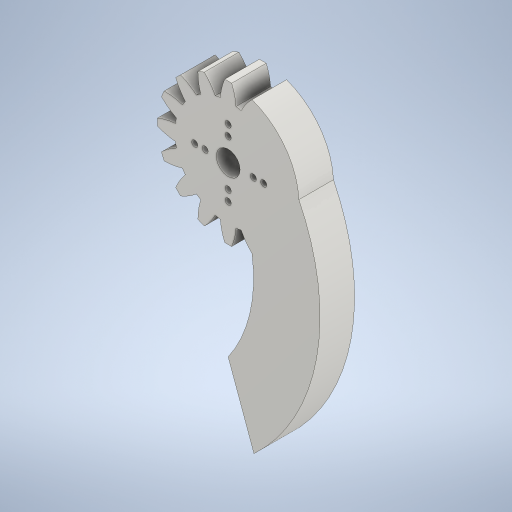
# Autodesk Inventor part: Spur Gear2
Saved by Autodesk Inventor 2024 (Build 280153000, 153)
## iProperties
CustomPartVersion: 0
Created: 2023-09-24
Part Number: Spur Gear2
Material: Steel
Document SubType Name: Modeling
Designer: jebes windows
Categories: <?xml version="1.0" encoding="UTF-16"?> <MemberInstance><Categories><FamilyTemplate><FamilyTemplateParameter ValueType="xs:double" Id="1" ObjectReferenceKey="da_z" ObjectType="kUserParameterObject"/><FamilyTemplateParameter ValueType="xs:double" Id="2" ObjectReferenceKey="da_b" ObjectType="kUserParameterObject"/><FamilyTemplateParameter ValueType="xs:double" Id="3" ObjectReferenceKey="da_beta" ObjectType="kUserParameterObject"/><FamilyTemplateParameter ValueType="xs:double" Id="4" ObjectReferenceKey="da_da" ObjectType="kUserParameterObject"/><FamilyTemplateParameter ValueType="xs:double" Id="5" ObjectReferenceKey="da_aw" ObjectType="kUserParameterObject"/><FamilyTemplateParameter ValueType="xs:string" Id="6" ObjectReferenceKey="EAIAABAAAACIAQAAAAAAAIAAAAAAAAAA" ObjectType="83910656" SubObjectId="SurfaceGeometry"/></FamilyTemplate><ParamToTemplateMap><ParamToTemplate CategoryParameter="//CategoryParameter[@InternalName='046C89C9-8512-4d59-83FE-43B91F4F132A']" TemplateParameter="1"/><ParamToTemplate CategoryParameter="//CategoryParameter[@InternalName='2552DF32-E462-4b46-AEBF-C6C7768E72AC']" TemplateParameter="2"/><ParamToTemplate CategoryParameter="//CategoryParameter[@InternalName='C9EE641D-15FC-4fae-A226-E94C4372FDD7']" TemplateParameter="3"/><ParamToTemplate><ParamToTemplate CategoryParameter="//CategoryParameter[@InternalName='00B6519A-459B-49c7-AD84-2E56D39A5744']" ConstantValue="0.102382"/></ParamToTemplate><ParamToTemplate><ParamToTemplate CategoryParameter="//CategoryParameter[@InternalName='04B31F0E-C7A6-4894-AA32-9629BEFACF47']" ConstantValue="1.000000"/></ParamToTemplate><ParamToTemplate><ParamToTemplate CategoryParameter="//CategoryParameter[@InternalName='43CBEC2E-7847-49e7-A936-2F7889FCB2D9']" ConstantValue="0.250000"/></ParamToTemplate><ParamToTemplate><ParamToTemplate CategoryParameter="//CategoryParameter[@InternalName='B1EFC894-105D-4ebd-86BF-FA20ED196853']" ConstantValue="0.302500"/></ParamToTemplate><ParamToTemplate><ParamToTemplate CategoryParameter="//CategoryParameter[@InternalName='51175063-3D10-4879-93E8-6246FE8B403D']" ConstantValue="2060000000.000000"/></ParamToTemplate><ParamToTemplate><ParamToTemplate CategoryParameter="//CategoryParameter[@InternalName='A3A52E27-4454-46a9-B0BD-C932399B70AF']" ConstantValue="0.300000"/></ParamToTemplate><ParamToTemplate><ParamToTemplate CategoryParameter="//CategoryParameter[@InternalName='91B76062-C214-41d9-B1B9-14D2AB99603D']" ConstantValue="0.150000"/></ParamToTemplate><ParamToTemplate><ParamToTemplate CategoryParameter="//CategoryParameter[@InternalName='374E806E-8B8A-4dda-A9AA-1039D6500AD2']" ConstantValue="6.666667"/></ParamToTemplate><ParamToTemplate><ParamToTemplate CategoryParameter="//CategoryParameter[@InternalName='2D373A89-B862-43d6-8D0B-0CBF12AB9F6C']" ConstantValue="0.349066"/></ParamToTemplate><ParamToTemplate CategoryParameter="//CategoryParameter[@InternalName='37777632-D6A2-4fac-9D53-DB8ACD95C989']" TemplateParameter="4"/><ParamToTemplate CategoryParameter="//CategoryParameter[@InternalName='FD1017F1-B727-4f7e-9707-0F86F1FF9423']" TemplateParameter="5"/><ParamToTemplate><ParamToTemplate CategoryParameter="//CategoryParameter[@InternalName='9E1B4470-B2D3-4ff1-B813-535BB4CDF51A']" ConstantValue="3520000.000000"/></ParamToTemplate><ParamToTemplate><ParamToTemplate CategoryParameter="//CategoryParameter[@InternalName='F8452263-BFF6-458c-9FB1-07C4B99E95CD']" ConstantValue="11400000.000000"/></ParamToTemplate><ParamToTemplate><ParamToTemplate CategoryParameter="//CategoryParameter[@InternalName='3E3BB259-FD49-497f-8171-6EBC954A3479']" ConstantValue="2.000000"/></ParamToTemplate><ParamToTemplate CategoryParameter="//CategoryParameter[@InternalName='27C3BAF2-7550-4e4b-AE2C-0DB134B7D9B7']" TemplateParameter="6"/></ParamToTemplateMap><Category DisplayName="Gear" InternalName="DC85795E-93AB-48d5-8EEE-5A27447B64BD" Mnemonic="Gear"><CategoryParameter DisplayName="z" InternalName="046C89C9-8512-4d59-83FE-43B91F4F132A" Mnemonic="z"/><CategoryParameter DisplayName="b" InternalName="2552DF32-E462-4b46-AEBF-C6C7768E72AC" Mnemonic="b"/><CategoryParameter DisplayName="||b|" InternalName="C9EE641D-15FC-4fae-A226-E94C4372FDD7" Mnemonic="beta"/><CategoryParameter DisplayName="x" InternalName="00B6519A-459B-49c7-AD84-2E56D39A5744" Mnemonic="x"/><CategoryParameter DisplayName="a*" InternalName="04B31F0E-C7A6-4894-AA32-9629BEFACF47" Mnemonic="a"/><CategoryParameter DisplayName="c*" InternalName="43CBEC2E-7847-49e7-A936-2F7889FCB2D9" Mnemonic="c"/><CategoryParameter DisplayName="r|.f|*" InternalName="B1EFC894-105D-4ebd-86BF-FA20ED196853" Mnemonic="rf"/><CategoryParameter DisplayName="E" InternalName="51175063-3D10-4879-93E8-6246FE8B403D" Mnemonic="E"/><CategoryParameter DisplayName="||m|" InternalName="A3A52E27-4454-46a9-B0BD-C932399B70AF" Mnemonic="mi"/><Category DisplayName="SpurGear" InternalName="26C5A22E-A91E-4dfd-A3B3-23CCAFAE1764" Mnemonic="SpurGear"><CategoryParameter DisplayName="m" InternalName="91B76062-C214-41d9-B1B9-14D2AB99603D" Mnemonic="m"/><CategoryParameter DisplayName="P" InternalName="374E806E-8B8A-4dda-A9AA-1039D6500AD2" Mnemonic="PP"/><CategoryParameter DisplayName="||a|" InternalName="2D373A89-B862-43d6-8D0B-0CBF12AB9F6C" Mnemonic="alpha"/><CategoryParameter DisplayName="d|.a|" InternalName="37777632-D6A2-4fac-9D53-DB8ACD95C989" Mnemonic="da"/><CategoryParameter DisplayName="a|.w|" InternalName="FD1017F1-B727-4f7e-9707-0F86F1FF9423" Mnemonic="aw"/><CategoryParameter DisplayName="||s||.Flim|" InternalName="9E1B4470-B2D3-4ff1-B813-535BB4CDF51A" Mnemonic="sFlim"/><CategoryParameter DisplayName="||s||.Hlim|" InternalName="F8452263-BFF6-458c-9FB1-07C4B99E95CD" Mnemonic="sHlim"/><CategoryParameter DisplayName="type" InternalName="3E3BB259-FD49-497f-8171-6EBC954A3479" Mnemonic="type"/><CategoryParameter DisplayName="PitchDiameter" InternalName="27C3BAF2-7550-4e4b-AE2C-0DB134B7D9B7" Mnemonic="IDS_PITCHDIAM"/></Category></Category></Categories></MemberInstance>
Density: 1 g/cm^3
Appearance: Steel
d16: 23,400 mm
d17: 0,000 mm
d41: 0,000 mm
d43: 23,400 mm
d46: 23,400 mm
d47: 0,000 mm
d48: 0,000 mm
Author: jebes windows
## iProperties of the stored document Spur Gear21_3DPrint.ipt
Created: 2023-09-24
Part Number: Spur Gear21_3DPrint
Material: Generic
Document SubType Name: Modeling
Designer: jebes windows
Density: 1 g/cm^3
Appearance: Default
Author: jebes windows
Autodesk Inventor part; units mm, degrees
ref_plane "YZ Plane" through (0, 0, 0) normal (1, 0, 0) x (0, 1, 0)
ref_plane "XZ Plane" through (0, 0, 0) normal (0, 1, 0) x (-1, 0, 0)
ref_plane "XY Plane" through (0, 0, 0) normal (0, 0, 1) x (1, 0, 0)
sketch "Sketch1" plane through (0, 0, 0) normal (0, 0, 1) x (1, 0, 0)
  circle A0 centre (0, 0) radius 13.65
  dimension "d0" = 27.3
  constraints: 1 centre point
  measures "d0" diameter of A0
extrude "Extrusion1" add sketch "Sketch1" along normal blind 6.6667
ref_plane "Work Plane2" through (0, 0, 3.3333) normal (0, 0, 1) x (1, 0, 0)
sketch "Sketch2" plane through (0, 0, 0) normal (0, 0, -1) x (-1, 0, 0)
  circle A0 centre (0, 0) radius 13.65 projected
  circle A1 centre (0, 0) radius 12
  dimension "d3" = 24
  constraints: 1 centre point, 1 coincident
  measures "d3" diameter of A1
surface extrude "Pitch Diameter" sketch "Sketch2" against normal through all shown no curves A1
ref_plane "Work Plane8" through (0, 0, 0) normal (0.9807853, 0.1950903, 0) x (0, 0, 1)
ref_plane "Work Plane9" through (0, 0, 0) normal (1, 0, 0) x (0, 1, 0)
spur gear teeth "Spur Gear" teeth 16 pitch diameter 24 tip diameter 27.3 root diameter 20.5571 face width 10 start plane through (0, 0, 0) normal (0, 0, -1) x (-1, 0, 0)
sketch "Sketch3" plane through (0, 0, 0) normal (0, 0, -1) x (-1, 0, 0)
  line L0 (1.9, -6.45) -> (1.9, -2.8797) projected
  arc A0 (1.9, -2.8797) -> (2.2091, -2.65) centre (0, 0) ccw projected
  line L1 (2.2091, -2.65) -> (14.1591, -1.997) projected
  arc A1 (14.1591, -1.997) -> (14.1591, 1.997) centre (14.05, 0) ccw projected
  line L2 (14.1591, 1.997) -> (2.2091, 2.65) projected
  arc A2 (2.2091, 2.65) -> (1.9, 2.8797) centre (0, 0) ccw projected
  line L3 (1.9, 2.8797) -> (1.9, 6.45) projected
  arc A3 (1.9, 6.45) -> (-1.9, 6.45) centre (0, 6.45) ccw projected
  line L4 (-1.9, 6.45) -> (-1.9, 3.2953) projected
  line L5 (-1.9, 3.2953) -> (-16.6263, 1.9922) projected
  arc A4 (-16.6263, 1.9922) -> (-16.6263, -1.9922) centre (-16.45, 0) ccw projected
  line L6 (-16.6263, -1.9922) -> (-1.9, -3.2953) projected
  line L7 (-1.9, -3.2953) -> (-1.9, -6.45) projected
  arc A5 (-1.9, -6.45) -> (1.9, -6.45) centre (0, -6.45) ccw projected
  circle A6 centre (-14.85, 0) radius 0.6 projected
  circle A7 centre (-16.85, 0) radius 0.6 projected
  circle A8 centre (-12.85, 0) radius 0.6 projected
  circle A9 centre (-10.85, 0) radius 0.6 projected
  circle A10 centre (-8.85, 0) radius 0.6 projected
  circle A11 centre (-6.85, 0) radius 0.6 projected
  circle A12 centre (-4.85, 0) radius 0.6 projected
  circle A13 centre (4.45, 0) radius 0.6 projected
  circle A14 centre (6.45, 0) radius 0.6 projected
  circle A15 centre (8.45, 0) radius 0.6 projected
  circle A16 centre (10.45, 0) radius 0.6 projected
  circle A17 centre (14.45, 0) radius 0.6 projected
  circle A18 centre (12.45, 0) radius 0.6 projected
  circle A19 centre (0, 0) radius 2.3 projected
  circle A20 centre (0, -4.45) radius 0.6 projected
  circle A21 centre (0, -6.45) radius 0.6 projected
  circle A22 centre (0, 4.45) radius 0.6 projected
  circle A23 centre (0, 6.45) radius 0.6 projected
  point P0 (0, 0)
extrude "Extrusion2" cut sketch "Sketch3" against normal blind 10 contours A11 | A12 | A13 | A14 | A19 | A20 | A21 | A22 | A23
sketch "Sketch4" plane through (0, 0, 6.6667) normal (0, 0, 1) x (1, 0, 0)
  circle A0 centre (0, 0) radius 2.3 projected
  circle A1 centre (0, 6.45) radius 0.6 projected
  circle A2 centre (0, -4.45) radius 0.6 projected
  circle A3 centre (-4.45, 0) radius 0.6 projected
  circle A4 centre (6.85, 0) radius 0.6 projected
  circle A5 centre (0, 4.45) radius 0.6 projected
  circle A6 centre (0, -6.45) radius 0.6 projected
  circle A7 centre (-6.45, 0) radius 0.6 projected
  circle A8 centre (4.85, 0) radius 0.6 projected
  arc A9 (-5.8361, 12.3395) -> (-5.2842, 8.8162) centre (5.1453, 12.2548) ccw projected
  arc A10 (-5.2842, 8.8162) -> (-6.1229, 8.2558) centre (0, 0) ccw projected
  arc A11 (-6.1229, 8.2558) -> (-9.1668, 10.114) centre (-13.2909, -0.0639) ccw projected
  arc A12 (-9.1668, 10.114) -> (-10.114, 9.1668) centre (0, 0) ccw projected
  arc A13 (-10.114, 9.1668) -> (-8.2558, 6.1229) centre (0.0639, 13.2909) ccw projected
  arc A14 (-8.2558, 6.1229) -> (-8.8162, 5.2842) centre (0, 0) ccw projected
  arc A15 (-8.8162, 5.2842) -> (-12.3395, 5.8361) centre (-12.2548, -5.1453) ccw projected
  arc A16 (-12.3395, 5.8361) -> (-12.8521, 4.5985) centre (0, 0) ccw projected
  arc A17 (-12.8521, 4.5985) -> (-9.9705, 2.4975) centre (-5.0272, 12.3037) ccw projected
  arc A18 (-9.9705, 2.4975) -> (-10.1673, 1.5082) centre (0, 0) ccw projected
  arc A19 (-10.1673, 1.5082) -> (-13.6336, 0.6698) centre (-9.3529, -9.4433) ccw projected
  arc A20 (-13.6336, 0.6698) -> (-13.6336, -0.6698) centre (0, 0) ccw projected
  arc A21 (-13.6336, -0.6698) -> (-10.1673, -1.5082) centre (-9.3529, 9.4433) ccw projected
  arc A22 (-10.1673, -1.5082) -> (-9.9705, -2.4975) centre (0, 0) ccw projected
  arc A23 (-9.9705, -2.4975) -> (-12.8521, -4.5985) centre (-5.0272, -12.3037) ccw projected
  arc A24 (-12.8521, -4.5985) -> (-12.3395, -5.8361) centre (0, 0) ccw projected
  arc A25 (-12.3395, -5.8361) -> (-8.8162, -5.2842) centre (-12.2548, 5.1453) ccw projected
  arc A26 (-8.8162, -5.2842) -> (-8.2558, -6.1229) centre (0, 0) ccw projected
  arc A27 (-8.2558, -6.1229) -> (-10.114, -9.1668) centre (0.0639, -13.2909) ccw projected
  arc A28 (-10.114, -9.1668) -> (-9.1668, -10.114) centre (0, 0) ccw projected
  arc A29 (-9.1668, -10.114) -> (-6.1229, -8.2558) centre (-13.2909, 0.0639) ccw projected
  arc A30 (-6.1229, -8.2558) -> (-5.2842, -8.8162) centre (0, 0) ccw projected
  arc A31 (-5.2842, -8.8162) -> (-5.8361, -12.3395) centre (5.1453, -12.2548) ccw projected
  arc A32 (-5.8361, -12.3395) -> (-4.5985, -12.8521) centre (0, 0) ccw projected
  arc A33 (-4.5985, -12.8521) -> (-2.4975, -9.9705) centre (-12.3037, -5.0272) ccw projected
  arc A34 (-2.4975, -9.9705) -> (-1.5082, -10.1673) centre (0, 0) ccw projected
  arc A35 (-1.5082, -10.1673) -> (-0.6698, -13.6336) centre (9.4433, -9.3529) ccw projected
  arc A36 (-0.6698, -13.6336) -> (0.6698, -13.6336) centre (0, 0) ccw projected
  arc A37 (0.6698, -13.6336) -> (1.5082, -10.1673) centre (-9.4433, -9.3529) ccw projected
  arc A38 (1.5082, -10.1673) -> (2.4975, -9.9705) centre (0, 0) ccw projected
  arc A39 (2.4975, -9.9705) -> (4.5985, -12.8521) centre (12.3037, -5.0272) ccw projected
  arc A40 (4.5985, -12.8521) -> (5.8361, -12.3395) centre (0, 0) ccw projected
  arc A41 (5.8361, -12.3395) -> (5.2842, -8.8162) centre (-5.1453, -12.2548) ccw projected
  arc A42 (5.2842, -8.8162) -> (6.1229, -8.2558) centre (0, 0) ccw projected
  arc A43 (6.1229, -8.2558) -> (9.1668, -10.114) centre (13.2909, 0.0639) ccw projected
  arc A44 (9.1668, -10.114) -> (10.114, -9.1668) centre (0, 0) ccw projected
  arc A45 (10.114, -9.1668) -> (8.2558, -6.1229) centre (-0.0639, -13.2909) ccw projected
  arc A46 (8.2558, -6.1229) -> (8.8162, -5.2842) centre (0, 0) ccw projected
  arc A47 (8.8162, -5.2842) -> (12.3395, -5.8361) centre (12.2548, 5.1453) ccw projected
  arc A48 (12.3395, -5.8361) -> (12.8521, -4.5985) centre (0, 0) ccw projected
  arc A49 (12.8521, -4.5985) -> (9.9705, -2.4975) centre (5.0272, -12.3037) ccw projected
  arc A50 (9.9705, -2.4975) -> (10.1673, -1.5082) centre (0, 0) ccw projected
  arc A51 (10.1673, -1.5082) -> (13.6336, -0.6698) centre (9.3529, 9.4433) ccw projected
  arc A52 (13.6336, -0.6698) -> (13.6336, 0.6698) centre (0, 0) ccw projected
  arc A53 (13.6336, 0.6698) -> (10.1673, 1.5082) centre (9.3529, -9.4433) ccw projected
  arc A54 (10.1673, 1.5082) -> (9.9705, 2.4975) centre (0, 0) ccw projected
  arc A55 (9.9705, 2.4975) -> (12.8521, 4.5985) centre (5.0272, 12.3037) ccw projected
  arc A56 (12.8521, 4.5985) -> (12.3395, 5.8361) centre (0, 0) ccw projected
  arc A57 (12.3395, 5.8361) -> (8.8162, 5.2842) centre (12.2548, -5.1453) ccw projected
  arc A58 (8.8162, 5.2842) -> (8.2558, 6.1229) centre (0, 0) ccw projected
  arc A59 (8.2558, 6.1229) -> (10.114, 9.1668) centre (-0.0639, 13.2909) ccw projected
  arc A60 (10.114, 9.1668) -> (9.1668, 10.114) centre (0, 0) ccw projected
  arc A61 (9.1668, 10.114) -> (6.1229, 8.2558) centre (13.2909, -0.0639) ccw projected
  arc A62 (6.1229, 8.2558) -> (5.2842, 8.8162) centre (0, 0) ccw projected
  arc A63 (5.2842, 8.8162) -> (5.8361, 12.3395) centre (-5.1453, 12.2548) ccw projected
  arc A64 (5.8361, 12.3395) -> (4.5985, 12.8521) centre (0, 0) ccw projected
  arc A65 (4.5985, 12.8521) -> (2.4975, 9.9705) centre (12.3037, 5.0272) ccw projected
  arc A66 (2.4975, 9.9705) -> (1.5082, 10.1673) centre (0, 0) ccw projected
  arc A67 (1.5082, 10.1673) -> (0.6698, 13.6336) centre (-9.4433, 9.3529) ccw projected
  arc A68 (0.6698, 13.6336) -> (-0.6698, 13.6336) centre (0, 0) ccw projected
  arc A69 (-0.6698, 13.6336) -> (-1.5082, 10.1673) centre (9.4433, 9.3529) ccw projected
  arc A70 (-1.5082, 10.1673) -> (-2.4975, 9.9705) centre (0, 0) ccw projected
  arc A71 (-2.4975, 9.9705) -> (-4.5985, 12.8521) centre (-12.3037, 5.0272) ccw projected
  arc A72 (-4.5985, 12.8521) -> (-5.8361, 12.3395) centre (0, 0) ccw projected
  line L0 (0, 0) -> (0, -50)
  circle A73 centre (-22.1184, -16.8796) radius 39.8269
  circle A74 centre (-22.1184, -16.8796) radius 27.0188
  circle A75 centre (0, 0) radius 13.65
  line L1 (0, -32.3971) -> (4.9764, -46.0696)
  point P0 (7.7779, 9.4337)
  point P1 (5.8113, 11.5125)
  point P2 (10.6741, 5.7221)
  point P3 (9.3146, 7.5776)
  point P4 (11.9378, 3.7689)
  point P5 (4.5985, -12.8521)
  point P6 (0, -32.3971)
  point P7 (-10.114, 9.1668)
  point P8 (-11.1829, 7.8273)
  point P9 (-8.5587, 6.4903)
  point P10 (-5.8361, 12.3395)
  point P11 (-9.1668, 10.114)
  point P12 (-0.6698, 13.6336)
  point P13 (-4.5985, 12.8521)
  point P14 (4.4956, 12.7494)
  point P15 (4.244, 12.9735)
  point P16 (0.6698, 13.6336)
  point P17 (13.6336, 0.6698)
  point P18 (12.8521, 4.5985)
  point P19 (12.3395, 5.8361)
  point P20 (10.114, 9.1668)
  point P21 (9.1668, 10.114)
  point P22 (5.8361, 12.3395)
  point P23 (4.5985, 12.8521)
  point P24 (12.8521, 4.5985)
  point P25 (12.3395, 5.8361)
  point P26 (10.114, 9.1668)
  point P27 (9.1668, 10.114)
  point P28 (5.8361, 12.3395)
  dimension "d53" = 54.0377
  dimension "d51" = 50
  dimension "d52" = 79.6539
  dimension "d61" = 20
  constraints: 4 end point, 3 point on circle, 1 centre point, 1 coincident, 1 point on line, 1 vertical, 6 other
  measures "d51" distance of L0.start L0.end
  measures "d52" diameter of A73
  measures "d61" angle of L0 L1
extrude "Extrusion3" add sketch "Sketch4" against normal blind 6.6667 contours A40 A75 A44 A48 A52 A73 L1 A74 | A41 A42 A43 A75 | A45 A46 A47 A75 | A53 A54 A55 A73 | A73 A55 A75 | A49 A50 A51 A75 | A73 A61 A62 A63 | A63 A75 A61 A73 | A73 A59 A75 A57 | A57 A58 A59 A73
equation "\"d0\" = da_da"
equation "\"d1\" = 0.666667 * da_b"
equation "\"d54\" = 0.666667 * da_b"
equation "\"d3\" = da_d"
equation "\"d16\" = da_aw"
equation "\"d43\" = da_aw"
equation "\"d46\" = da_aw"
equation "\"da_da\" = 27.3"
equation "\"da_b\" = 10"
equation "\"da_d\" = 24"
equation "\"da_aw\" = 23.4"
body "Solid1"
body "Srf1"
